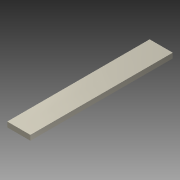
# Autodesk Inventor part: Piezoelectric_Element
Saved by Autodesk Inventor 2011 SP2 (Build 150309200, 309)
## iProperties
Created: 2011-09-20
Part Number: Piezoelectric_Element
Document SubType Name: Modeling
Designer: sungwook
Density: 7.7 g/cm^3
Material: PZT
Author: sungwook
Autodesk Inventor part; units mm, degrees
ref_plane "YZ Plane" through (0, 0, 0) normal (1, 0, 0) x (0, 1, 0)
ref_plane "XZ Plane" through (0, 0, 0) normal (0, 1, 0) x (-1, 0, 0)
ref_plane "XY Plane" through (0, 0, 0) normal (0, 0, 1) x (1, 0, 0)
sketch "Sketch1" plane through (0, 0, 0) normal (0, 0, 1) x (1, 0, 0)
  line L0 (-0.485, 2.985) -> (0.485, 2.985)
  line L1 (0.485, 2.985) -> (0.485, -2.985)
  line L2 (0.485, -2.985) -> (-0.485, -2.985)
  line L3 (-0.485, -2.985) -> (-0.485, 2.985)
  point P0 (0, 0)
  point P1 (0, 2.985)
  point P2 (0.485, 0)
  dimension "d0" = 0.97
  dimension "d1" = 5.97
  constraints: 8 end point, 2 midpoint, 2 parallel, 1 horizontal, 1 horizontal alignment, 1 perpendicular, 1 vertical alignment
  measures "d0" distance of L0.start L0.end
  measures "d1" distance of L0.end L1.end
extrude "Extrusion1" add sketch "Sketch1" along normal blind 0.21
body "Solid1"
